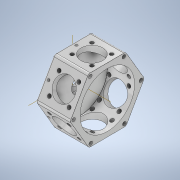
# Autodesk Inventor part: crank case
Saved by Autodesk Inventor 2021.1 (Build 251245000, 245)
## iProperties
Created: 2020-08-29
Part Number: crank case
Material: Aluminum 6061
Document SubType Name: Sheet Metal
Designer: Vamshi
Density: 2.7 g/cm^3
Sheet Metal Rule: Default
Appearance: Aluminum - Polished
Mass: 8625.86 g
Surface Area: 3573.59 cm^2
Volume: 3194.76 cm^3
Author: Vamshi
Autodesk Inventor part; units mm, degrees
ref_plane "YZ Plane" through (0, 0, 0) normal (1, 0, 0) x (0, 1, 0)
ref_plane "XZ Plane" through (0, 0, 0) normal (0, 1, 0) x (-1, 0, 0)
ref_plane "XY Plane" through (0, 0, 0) normal (0, 0, 1) x (1, 0, 0)
sketch "Sketch1" plane through (0, 0, 0) normal (0, 0, 1) x (1, 0, 0)
  line L0 (71.3654, -134.1058) -> (-69.412, -135.1271)
  line L1 (-80.4563, -128.8571) -> (-151.7295, -7.451)
  line L2 (-151.8217, 5.2487) -> (-82.3175, 127.6761)
  line L3 (-71.3654, 134.1058) -> (69.412, 135.1271)
  line L4 (80.4563, 128.8571) -> (151.7295, 7.451)
  line L5 (151.8217, -5.2487) -> (82.3175, -127.6761)
  arc A0 (-71.3654, 134.1058) -> (-82.3175, 127.6761) centre (-71.2732, 121.4061) ccw
  arc A1 (80.4563, 128.8571) -> (69.412, 135.1271) centre (69.5041, 122.4275) ccw
  arc A2 (151.8217, -5.2487) -> (151.7295, 7.451) centre (140.7774, 1.0214) ccw
  arc A3 (71.3654, -134.1058) -> (82.3175, -127.6761) centre (71.2732, -121.4061) ccw
  arc A4 (-80.4563, -128.8571) -> (-69.412, -135.1271) centre (-69.5041, -122.4275) ccw
  arc A5 (-151.8217, 5.2487) -> (-151.7295, -7.451) centre (-140.7774, -1.0214) ccw
  point P0 (0, 0)
  point P1 (0, 0)
  point P2 (78.6975, -134.0526)
  point P3 (-76.7442, -135.1803)
  point P4 (-155.4417, -1.1278)
  point P5 (-78.6975, 134.0526)
  point P6 (76.7442, 135.1803)
  point P7 (155.4417, 1.1278)
  dimension "d0" = 269.24
  dimension "d1" = 12.7
  constraints: 12 end point, 12 point on circle, 12 point on line, 12 tangent, 6 centre point, 5 equal radius, 1 coincident, 13 other
  measures "d0" distance between parallel lines of L0 L3
  measures "d1" radius of A0
extrude "Extrusion1" add sketch "Sketch1" along normal blind 144.78
sketch "Sketch2" plane through (0, 0, 144.78) normal (0, 0, 1) x (1, 0, 0)
  circle A0 centre (0, 0) radius 114.3
  dimension "d4" = 228.6
  constraints: 1 centre point, 1 coincident
  measures "d4" diameter of A0
extrude "Extrusion2" cut sketch "Sketch2" against normal blind 114.3
chamfer "Chamfer1" distance 0.508 angle 45 1 edges at (-114.3, 0, 30.48) measured on face at (-5.7855, 21.5918, 30.48)
sketch "Sketch6" plane through (0, 0, 144.78) normal (0, 0, 1) x (1, 0, 0)
  arc A0 (80.4563, 128.8571) -> (69.412, 135.1271) centre (69.5041, 122.4275) ccw projected
  circle A1 centre (69.5041, 122.4275) radius 7.62
  circle A2 centre (-71.2732, 121.4061) radius 7.62
  circle A3 centre (-140.7774, -1.0214) radius 7.62
  circle A4 centre (-69.5041, -122.4275) radius 7.62
  circle A5 centre (71.2732, -121.4061) radius 7.62
  circle A6 centre (140.7774, 1.0214) radius 7.62
  point P0 (0, 0)
  dimension "d10" = 15.24
  dimension "d13" = 360
  constraints: 6 centre point, 1 coincident, 13 other
  measures "d10" diameter of A1
extrude "Extrusion3" cut sketch "Sketch6" against normal blind 30.48
sketch "Sketch7" plane through (-71.3654, 134.1058, 144.78) normal (-0.0072551, 0.9999737, 0) x (0.9999737, 0.0072551, 0)
  circle A0 centre (70.3905, 63.5) radius 45.72
  line L0 (140.7811, 0) -> (0, 0) projected
  line L1 (140.7811, 144.78) -> (0, 144.78) projected
  point P0 (70.3905, 144.78)
  point P1 (70.3905, 144.78)
  dimension "d17" = 91.44
  dimension "d18" = 63.5
  constraints: 1 centre point, 1 midpoint, 1 vertical alignment
  measures "d17" diameter of A0
  measures "d18" distance from line of L0 A0.centre
extrude "Extrusion4" cut sketch "Sketch7" against normal up to surface
pattern_circular "Circular Pattern1" count 6 over 360 about axis through (0, 0, 144.78) along (0, 0, -1) of "Extrusion4"
thread "Thread1" size "5/8-11 UNC" class "2B" standard "ANSI Unified Screw Threads" full length
thread "Thread2" size "5/8-11 UNC" class "2B" standard "ANSI Unified Screw Threads" full length
thread "Thread3" size "5/8-11 UNC" class "2B" standard "ANSI Unified Screw Threads" full length
thread "Thread4" size "5/8-11 UNC" class "2B" standard "ANSI Unified Screw Threads" full length
thread "Thread5" size "5/8-11 UNC" class "2B" standard "ANSI Unified Screw Threads" full length
thread "Thread6" size "5/8-11 UNC" class "2B" standard "ANSI Unified Screw Threads" full length
thread "Thread7" size "5/8-11 UNC" class "2B" standard "ANSI Unified Screw Threads" full length
sketch "Sketch8" plane through (-71.3654, 134.1058, 144.78) normal (-0.0072551, 0.9999737, 0) x (0.9999737, 0.0072551, 0)
  circle A0 centre (70.3905, 63.5) radius 45.72 construction
  circle A1 centre (70.3905, 63.5) radius 58.42 construction
  line L0 (70.3905, 144.78) -> (70.3905, 0) construction
  line L1 (184.6905, 0) -> (-43.9095, 0) construction
  line L2 (70.3905, 63.5) -> (140.7811, 63.5) construction
  line L3 (140.7811, 144.78) -> (140.7811, 0) construction
  line L4 (70.3905, 63.5) -> (11.9705, 63.5) construction
  line L5 (70.3905, 63.5) -> (124.4866, 117.5961) construction
  circle A2 centre (111.6997, 104.8092) radius 7.62
  circle A3 centre (29.0814, 104.8092) radius 7.62
  circle A4 centre (29.0814, 22.1908) radius 7.62
  circle A5 centre (111.6997, 22.1908) radius 7.62
  dimension "d38" = 116.84
  dimension "d39" = 45
  dimension "d40" = 15.24
  dimension "d43" = 360
  constraints: 8 end point, 5 centre point, 2 point on circle, 2 point on line, 1 coincident, 1 midpoint, 1 perpendicular, 9 other
  measures "d38" diameter of A1
  measures "d39" angle of L2 L5
  measures "d40" diameter of A2
extrude "Extrusion5" cut sketch "Sketch8" against normal up to surface
pattern_circular "Circular Pattern2" count 6 over 360 about axis through (0, 0, 144.78) along (0, 0, -1) of "Extrusion5"
thread "Thread8" size "5/8-11 UNC" class "2B" standard "ANSI Unified Screw Threads" full length
thread "Thread9" size "5/8-11 UNC" class "2B" standard "ANSI Unified Screw Threads" full length
thread "Thread10" size "5/8-11 UNC" class "2B" standard "ANSI Unified Screw Threads" full length
thread "Thread11" size "5/8-11 UNC" class "2B" standard "ANSI Unified Screw Threads" full length
thread "Thread12" size "5/8-11 UNC" class "2B" standard "ANSI Unified Screw Threads" full length
thread "Thread13" size "5/8-11 UNC" class "2B" standard "ANSI Unified Screw Threads" full length
thread "Thread14" size "5/8-11 UNC" class "2B" standard "ANSI Unified Screw Threads" full length
thread "Thread15" size "5/8-11 UNC" class "2B" standard "ANSI Unified Screw Threads" full length
thread "Thread16" size "5/8-11 UNC" class "2B" standard "ANSI Unified Screw Threads" full length
thread "Thread17" size "5/8-11 UNC" class "2B" standard "ANSI Unified Screw Threads" full length
thread "Thread18" size "5/8-11 UNC" class "2B" standard "ANSI Unified Screw Threads" full length
thread "Thread19" size "5/8-11 UNC" class "2B" standard "ANSI Unified Screw Threads" full length
thread "Thread20" size "5/8-11 UNC" class "2B" standard "ANSI Unified Screw Threads" full length
thread "Thread21" size "5/8-11 UNC" class "2B" standard "ANSI Unified Screw Threads" full length
thread "Thread22" size "5/8-11 UNC" class "2B" standard "ANSI Unified Screw Threads" full length
thread "Thread23" size "5/8-11 UNC" class "2B" standard "ANSI Unified Screw Threads" full length
thread "Thread24" size "5/8-11 UNC" class "2B" standard "ANSI Unified Screw Threads" full length
thread "Thread25" size "5/8-11 UNC" class "2B" standard "ANSI Unified Screw Threads" full length
thread "Thread26" size "5/8-11 UNC" class "2B" standard "ANSI Unified Screw Threads" full length
thread "Thread27" size "5/8-11 UNC" class "2B" standard "ANSI Unified Screw Threads" full length
thread "Thread28" size "5/8-11 UNC" class "2B" standard "ANSI Unified Screw Threads" full length
thread "Thread29" size "5/8-11 UNC" class "2B" standard "ANSI Unified Screw Threads" full length
thread "Thread30" size "5/8-11 UNC" class "2B" standard "ANSI Unified Screw Threads" full length
thread "Thread31" size "5/8-11 UNC" class "2B" standard "ANSI Unified Screw Threads" full length
thread "Thread32" size "5/8-11 UNC" class "2B" standard "ANSI Unified Screw Threads" full length
thread "Thread33" size "5/8-11 UNC" class "2B" standard "ANSI Unified Screw Threads" full length
thread "Thread34" size "5/8-11 UNC" class "2B" standard "ANSI Unified Screw Threads" full length
thread "Thread35" size "5/8-11 UNC" class "2B" standard "ANSI Unified Screw Threads" full length
thread "Thread36" size "5/8-11 UNC" class "2B" standard "ANSI Unified Screw Threads" full length
thread "Thread37" size "5/8-11 UNC" class "2B" standard "ANSI Unified Screw Threads" full length
thread "Thread38" size "5/8-11 UNC" class "2B" standard "ANSI Unified Screw Threads" full length
fillet "Fillet1" radius 5.08 12 edges at (-77.7029, 132.3583, 0) (-117.0696, 66.4624, 0) (-153.4771, -1.1135, 0) (-116.0929, -68.1541, 0) (-75.7742, -133.4718, 0) (0.9767, -134.6165, 0) (77.7029, -132.3583, 0) (117.0696, -66.4624, 0) (153.4771, 1.1135, 0) (116.0929, 68.1541, 0) (75.7742, 133.4718, 0) (-0.9767, 134.6165, 0)
sketch "Sketch9" plane through (0, 0, 30.48) normal (0, 0, 1) x (1, 0, 0)
  circle A0 centre (0, 0) radius 35.56
  circle A1 centre (0, 0) radius 17.78
  dimension "d113" = 71.12
  dimension "d114" = 35.56
  constraints: 2 centre point, 2 coincident
  measures "d113" diameter of A0
  measures "d114" diameter of A1
extrude "Extrusion6" cut sketch "Sketch9" against normal blind 20.32 contours A0 | A1
extrude "Extrusion7" cut sketch "Sketch9" against normal through all contours A1
sketch "Sketch10" plane through (-71.3654, 134.1058, 144.78) normal (-0.0072551, 0.9999737, 0) x (0.9999737, 0.0072551, 0)
  circle A0 centre (70.3905, 128.1671) radius 5.08
  point P0 (70.3905, 144.78)
  dimension "d119" = 10.16
  constraints: 1 centre point
  measures "d119" diameter of A0
extrude "Extrusion8" cut sketch "Sketch10" against normal blind 91.44
pattern_circular "Circular Pattern3" count 6 over 360 about axis through (0, 0, 144.78) along (0, 0, -1) of "Extrusion8"
sketch "Sketch11" plane through (0, 0, 0) normal (0, 0, -1) x (-1, 0, 0)
  circle A0 centre (0, 50.8) radius 5.08
  point P0 (0, 0)
  dimension "d125" = 10.16
  dimension "d126" = 50.8
  constraints: 1 centre point, 1 vertical alignment
  measures "d125" diameter of A0
  measures "d126" distance of point (0, 0) A0.centre
extrude "Extrusion9" cut sketch "Sketch11" against normal blind 20.32
pattern_circular "Circular Pattern4" count 6 over 360 about axis through (0, 0, 30.48) along (0, 0, -1) of "Extrusion9"
chamfer "Chamfer2" distance 0.254 angle 45 12 edges at (-0.9767, 134.6165, 144.78) (-77.7029, 132.3583, 144.78) (-117.0696, 66.4624, 144.78) (-153.4771, -1.1135, 144.78) (-116.0929, -68.1541, 144.78) (-75.7742, -133.4718, 144.78) (0.9767, -134.6165, 144.78) (77.7029, -132.3583, 144.78) (117.0696, -66.4624, 144.78) (153.4771, 1.1135, 144.78) (116.0929, 68.1541, 144.78) (75.7742, 133.4718, 144.78)
equation "\"GapSize\" = Thickness"
equation "\"BendRadius\" = Thickness"
equation "\"MinimumRemnant\" = 2 * Thickness"
equation "\"BendReliefDepth\" = 0.5 * Thickness"
equation "\"BendReliefWidth\" = Thickness"
equation "\"CornerReliefSize\" = 4 * Thickness"
equation "\"JacobiRadiusSize\" = BendRadius"
equation "\"TransitionRadius\" = BendRadius"
equation "\"Thickness\" = 3.048"
body "Solid1"
